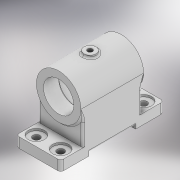
# Autodesk Inventor part: 支座
Saved by Autodesk Inventor 2020 (Build 240168000, 168)
## iProperties
Created: 2021-03-29
Part Number: 支座
Material: 常规
Document SubType Name: Modeling
Designer: 唐晨超
Density: 1 g/cm^3
Appearance: 默认
Author: 唐晨超
Title: 支座
Autodesk Inventor part; units mm, degrees
ref_plane "YZ Plane" through (0, 0, 0) normal (1, 0, 0) x (0, 1, 0)
ref_plane "XZ Plane" through (0, 0, 0) normal (0, 1, 0) x (-1, 0, 0)
sketch "草图1" plane through (0, 0, 0) normal (0, 1, 0) x (-1, 0, 0)
  line L0 (0, 0) -> (0, -51) construction
  line L1 (0, -51) -> (22, -51)
  line L2 (22, -51) -> (22, 51)
  line L3 (22, 51) -> (-22, 51)
  line L4 (-22, 51) -> (-22, -51)
  line L5 (-22, -51) -> (0, -51)
  dimension "d0" = 51
  dimension "d1" = 22
  dimension "d2" = 102
  dimension "d3" = 44
  dimension "d4" = 102
  constraints: 12 end point, 3 perpendicular, 2 vertical
  measures "d0" distance of L0.start L0.end
  measures "d1" distance of L0.end L1.end
  measures "d2" distance of L1.end L2.end
  measures "d3" distance of L2.end L3.end
  measures "d4" distance of L3.end L4.end
extrude "拉伸1" add sketch "草图1" against normal blind 10
sketch "草图2" plane through (0, -10, 0) normal (0, -1, 0) x (1, 0, 0)
  line L0 (16, 0) -> (16, 23)
  line L1 (16, 23) -> (-16, 23)
  line L2 (-16, 23) -> (-16, -23)
  line L3 (-16, -23) -> (16, -23)
  line L4 (16, -23) -> (16, 0)
  point P0 (0, 0)
  dimension "d9" = 16
  dimension "d10" = 23
  dimension "d11" = 32
  dimension "d12" = 46
  dimension "d13" = 32
  constraints: 10 end point, 2 perpendicular, 1 point on line
  measures "d9" distance of point (0, 0) L0.start
  measures "d10" distance of L0.start L0.end
  measures "d11" distance of L0.end L1.end
  measures "d12" distance of L1.end L2.end
  measures "d13" distance of L2.end L3.end
sketch "草图3" plane through (0, 0, 0) normal (0, 1, 0) x (1, 0, 0)
  line L0 (-22, 51) -> (-22, -51) projected
  line L1 (22, -51) -> (22, 51) projected
  line L2 (0, -29) -> (-22, -29)
  line L3 (-22, -29) -> (22, -29)
  line L4 (22, -29) -> (22, 29)
  line L5 (22, 29) -> (-22, 29)
  line L6 (-22, 29) -> (-22, -29)
  point P0 (0, 0)
  dimension "d16" = 29
  dimension "d17" = 58
  constraints: 10 end point, 2 parallel, 2 perpendicular, 2 point on line, 1 horizontal
  measures "d16" distance of point (0, 0) L2.start
  measures "d17" distance of L4.end L3.end
extrude "拉伸5" cut sketch "草图2" against normal blind 24
sketch "草图4" plane through (0, 0, 0) normal (0, 0, 1) x (1, 0, 0)
  line L0 (-22, -10) -> (22, -10) projected
  line L1 (0, -10) -> (0, 34) construction
  circle A0 centre (0, 34) radius 17
  circle A1 centre (0, 34) radius 15
  circle A2 centre (0, 34) radius 22
  point P0 (0, 0)
  dimension "d24" = 44
  dimension "d25" = 34
  dimension "d26" = 30
  dimension "d27" = 44
  constraints: 3 centre point, 3 coincident, 2 end point, 1 midpoint, 1 vertical
  measures "d24" distance of L1.start L1.end
  measures "d25" diameter of A0
  measures "d26" diameter of A1
  measures "d27" diameter of A2
extrude "拉伸6" add sketch "草图4" along normal mid plane 62 contours A0 | A2
extrude "拉伸7" add sketch "草图3" along normal up to surface round surface about axis through (0, 34, 0) along (0, 0, 1) radius 22 far side no
sketch "草图5" plane through (0, 0, 0) normal (0, 0, 1) x (1, 0, 0)
  circle A0 centre (0, 34) radius 15 projected
  circle A1 centre (0, 34) radius 17
  point P0 (0, 0)
  dimension "d32" = 34
  constraints: 1 centre point, 1 coincident
  measures "d32" diameter of A1
extrude "拉伸8" cut sketch "草图5" along normal mid plane 32 contours A0 | A1
ref_plane "工作平面1" through (0, 56, 0) normal (0, -1, 0) x (1, 0, 0)
sketch "草图8" plane through (0, 0, 0) normal (0, 1, 0) x (1, 0, 0)
  line L0 (22, 51) -> (-22, 51) projected
  line L1 (-22, 51) -> (-22, 29) projected
  line L2 (-22, -51) -> (-22, 51) projected
  line L3 (-22, 51) -> (-22, 41)
  line L4 (-22, 41) -> (-12, 41) construction
  line L5 (0, 51) -> (0, -51) construction
  line L6 (22, -51) -> (-22, -51) projected
  line L7 (22, 0) -> (-22.9774, 0) construction
  line L8 (-22, 0) -> (22.9774, 0) construction
  point P0 (0, 0)
  point P1 (12, 41)
  point P2 (-12, -41)
  point P3 (-12, -41)
  point P4 (12, -41)
  dimension "d42" = 10
  dimension "d43" = 10
  constraints: 10 end point, 6 symmetric about line, 2 coincident, 2 midpoint, 1 horizontal, 1 perpendicular, 1 point on line
  measures "d42" distance of L0.end L3.end
  measures "d43" distance of L3.end L4.end
hole "孔2" at (12, 0, -41) at (-12, 0, -41) at (-12, 0, 41) at (12, 0, 41) direction (0, -1, 0) diameter 16 depth 2
hole "孔3" at (12, 0, -41) at (-12, 0, -41) at (-12, 0, 41) at (12, 0, 41) direction (0, -1, 0) diameter 7 end through all
fillet "圆角1" radius 3 4 edges at (-22, -5, -51) (22, -5, -51) (-22, -5, 51) (22, -5, 51)
sketch "草图9" plane through (0, 56, 0) normal (0, -1, 0) x (1, 0, 0)
  circle A0 centre (0, 0) radius 3
  dimension "d60" = 6
  constraints: 1 centre point, 1 coincident
  measures "d60" diameter of A0
sketch "草图10" plane through (0, 0, 0) normal (0, -1, 0) x (1, 0, 0)
  line L0 (-16, 23) -> (-16, -23) projected
  line L1 (-16, -23) -> (16, -23) projected
  line L2 (16, -23) -> (16, 23) projected
  line L3 (16, 23) -> (-16, 23) projected
  line L4 (-16, 23) -> (16, 23) projected
  line L5 (16, 23) -> (-16, 23)
  line L6 (-16, 23) -> (-16, -23)
  line L7 (-16, -23) -> (16, -23)
  line L8 (16, -23) -> (16, 23)
  point P0 (0, 0)
  constraints: 8 end point, 2 parallel, 1 horizontal, 1 perpendicular
extrude "拉伸10" cut sketch "草图10" against normal up to surface round surface about axis through (0, 34, 0) along (0, 0, 1) radius 22 far side no
sketch "草图11" plane through (-22, -10, 48) normal (-1, 0, 0) x (0, 0, 1)
  line L0 (0, 0) -> (-96, 0) projected
  line L1 (-71, 0) -> (-25, 0) projected
  line L2 (-48, 0) -> (-25, 0)
  line L3 (-25, 0) -> (-25, 3)
  line L4 (-25, 3) -> (-71, 3)
  line L5 (-71, 3) -> (-71, 0)
  line L6 (-71, 0) -> (-48, 0)
  point P0 (-48, 10)
  dimension "d66" = 23
  dimension "d67" = 3
  dimension "d68" = 46
  constraints: 10 end point, 2 perpendicular, 2 point on line, 1 collinear, 1 midpoint, 1 parallel
  measures "d66" distance of L2.start L2.end
  measures "d67" distance of L2.end L3.end
  measures "d68" distance of L3.end L4.end
extrude "拉伸11" cut sketch "草图11" against normal through all
sketch "草图12" plane through (0, 56, 0) normal (0, -1, 0) x (1, 0, 0)
  circle A0 centre (0, 0) radius 6
  dimension "d73" = 12
  constraints: 1 centre point, 1 coincident
  measures "d73" diameter of A0
extrude "拉伸12" add sketch "草图12" against normal blind 2
extrude "拉伸13" add sketch "草图12" along normal blind 2
sketch "草图13" plane through (0, 58, 0) normal (0, 1, 0) x (1, 0, 0)
  circle A0 centre (0, 0) radius 6 projected
  constraints: 1 coincident
hole "孔4" at (0, 58, 0) direction (0, -1, 0) diameter 4.917 end up to surface thread size "M6x1" designation "M6" class "6H" standard "GB Metric profile"
fillet "圆角6" radius 2 4 edges at (4.5747, 55.5191, 3.8823) (4.5814, 55.5177, -3.8743) (-4.5811, 55.5178, 3.8748) (-4.5747, 55.5191, -3.8823)
fillet "圆角7" radius 2 2 edges at (0, 12, -29) (0, 12, 29)
fillet "圆角8" radius 2 4 edges at (22, -7, 0) (16, -7, 0) (-16, -7, 0) (-22, -7, 0)
fillet "圆角9" radius 2 2 edges at (-17, 34, 16) (-17, 34, -16)
fillet "圆角10" radius 2 8 edges at (-22, 29.258, -29.6712) (-22, 12.2042, -29) (22, 29.258, -29.6712) (22, 12.2042, -29) (-22, 29.258, 29.6712) (-22, 12.2042, 29) (22, 29.258, 29.6712) (22, 12.2042, 29)
